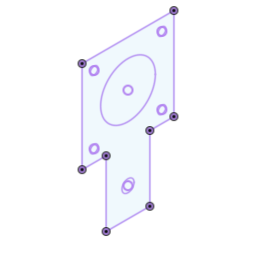
motor_mount (Autodesk Fusion 360 design; units mm, degrees)
Autodesk Fusion 360 part; units mm, degrees
sketch "Sketch1" plane through (0, 0, 0) normal (1, 0, 0) x (0, 0, -1)
  line L0 (-4, 70) -> (-4, -60) construction
  line L1 (-65, 8) -> (55, 8) construction
  line L2 (-25, 50) -> (17, 50)
  line L3 (17, 50) -> (17, 8)
  line L4 (17, 8) -> (-25, 8)
  line L5 (-25, 8) -> (-25, 50)
  line L6 (-14, 8) -> (6, 8)
  line L7 (6, 8) -> (6, -22)
  line L8 (6, -22) -> (-14, -22)
  line L9 (-14, -22) -> (-14, 8)
  line L10 (-25, 29) -> (17, 29) construction
  circle A0 centre (-19.5, 44.5) radius 1.75
  circle A1 centre (11.5, 44.5) radius 1.75
  circle A2 centre (-19.5, 13.5) radius 1.75
  circle A3 centre (11.5, 13.5) radius 1.75
  circle A4 centre (-4, 29) radius 12.5
  circle A5 centre (-4, -8.8575) radius 2.75
  dimension "d1" = 42
  dimension "d2" = 20
  dimension "d3" = 30
  dimension "d4" = 42
  dimension "d5" = 3.5
  dimension "d6" = 15.5
  dimension "d7" = 15.5
  dimension "d8" = 25
  dimension "d9" = 5.5
  constraint vertical L0
  constraint horizontal L1
  constraint horizontal L2
  constraint vertical L3
  constraint horizontal L4
  constraint vertical L5
  constraint coincident L1 L3.end
  constraint horizontal L6
  constraint vertical L7
  constraint horizontal L8
  constraint vertical L9
  constraint coincident L1 L6.start
  constraint symmetric L0 L3 L5
  constraint symmetric L0 L7 L9
  constraint midpoint L5 L10.start
  constraint midpoint L3 L10.end
  constraint symmetric L0 A0 A1
  constraint symmetric L10 A0 A2
  constraint symmetric L10 A1 A3
  constraint midpoint L10 A4.centre
  constraint coincident L0 A5.centre
  measures "d1" distance of L2.start L2.end
  measures "d2" distance of L7.end L8.end
  measures "d3" distance of L6.end L7.end
  measures "d4" distance of L2.end L3.end
  measures "d5" diameter of A0
  measures "d6" distance of L0 A0.centre
  measures "d7" distance of L10 A0.centre
  measures "d8" diameter of A4
  measures "d9" diameter of A5
extrude "Extrude1" add sketch "Sketch1" along normal blind 6
sketch "Sketch3" plane through (6, 0, 0) normal (1, 0, 0) x (0, 0, -1)
  circle A0 centre (-4, 29) radius 12.5
  circle A1 centre (-19.5, 44.5) radius 1.75
  circle A2 centre (11.5, 13.5) radius 1.75
  circle A3 centre (-19.5, 13.5) radius 1.75
  circle A4 centre (11.5, 44.5) radius 1.75
  circle A5 centre (-4, -8.8575) radius 2.75
  line L0 (-14, -22) -> (6, -22)
  line L1 (6, -22) -> (6, 8)
  line L2 (6, 8) -> (17, 8)
  line L3 (17, 8) -> (17, 50)
  line L4 (17, 50) -> (-25, 50)
  line L5 (-25, 50) -> (-25, 8)
  line L6 (-25, 8) -> (-14, 8)
  line L7 (-14, 8) -> (-14, -22)
hidden bodies 1
